Autodesk Inventor part; units mm, degrees
(part 2 of 3)
  spline S217 degree 2 poles (-31.2508, 23.9795) (-31.8051, 23.9795) (-32.4202, 24.6213) (-32.4202, 25.1805) knots 0 0 0 1 2 2 2
  spline S218 degree 2 poles (-32.4202, 25.1805) (-32.4202, 25.7445) (-31.8051, 26.3839) (-31.2508, 26.3839) knots 0 0 0 1 2 2 2
  spline S219 degree 2 poles (-31.2508, 26.3839) (-30.6965, 26.3839) (-30.0839, 25.7421) (-30.0839, 25.1805) knots 0 0 0 1 2 2 2
  spline S220 degree 2 poles (-30.8059, 25.1756) (-30.8059, 25.3774) (-30.8716, 25.6472) (-30.9299, 25.7275) knots 0 0 0 1 2 2 2
  spline S221 degree 2 poles (-30.9299, 25.7275) (-30.9931, 25.8126) (-31.1511, 25.8782) (-31.2508, 25.8782) knots 0 0 0 1 2 2 2
  spline S222 degree 2 poles (-31.2508, 25.8782) (-31.3481, 25.8782) (-31.5012, 25.8199) (-31.5644, 25.7372) knots 0 0 0 1 2 2 2
  spline S223 degree 2 poles (-31.5644, 25.7372) (-31.6252, 25.6594) (-31.6981, 25.3847) (-31.6981, 25.1756) knots 0 0 0 1 2 2 2
  spline S224 degree 2 poles (-31.6981, 25.1756) (-31.6981, 24.969) (-31.6301, 24.7137) (-31.5741, 24.6359) knots 0 0 0 1 2 2 2
  spline S225 degree 2 poles (-31.5741, 24.6359) (-31.5182, 24.5581) (-31.3481, 24.4852) (-31.2459, 24.4852) knots 0 0 0 1 2 2 2
  spline S226 degree 2 poles (-31.2459, 24.4852) (-31.1609, 24.4852) (-30.9858, 24.5581) (-30.9323, 24.631) knots 0 0 0 1 2 2 2
  spline S227 degree 2 poles (-30.9323, 24.631) (-30.8716, 24.7161) (-30.8059, 24.9617) (-30.8059, 25.1756) knots 0 0 0 1 2 2 2
  line L287 (-29.0045, 24.05) -> (-29.7095, 24.05)
  line L288 (-29.7095, 24.05) -> (-29.7095, 27.1837)
  line L289 (-29.7095, 27.1837) -> (-29.0045, 27.1837)
  line L290 (-29.0045, 27.1837) -> (-29.0045, 24.05)
  line L291 (15.1937, 24.05) -> (14.4449, 24.05)
  line L292 (14.4449, 24.05) -> (14.4449, 26.0387)
  line L293 (14.4449, 26.0387) -> (13.9003, 24.755)
  line L294 (13.9003, 24.755) -> (13.3849, 24.755)
  line L295 (13.3849, 24.755) -> (12.8404, 26.0387)
  line L296 (12.8404, 26.0387) -> (12.8404, 24.05)
  line L297 (12.8404, 24.05) -> (12.1305, 24.05)
  line L298 (12.1305, 24.05) -> (12.1305, 27.05)
  line L299 (12.1305, 27.05) -> (12.9984, 27.05)
  line L300 (12.9984, 27.05) -> (13.6645, 25.5694)
  line L301 (13.6645, 25.5694) -> (14.3258, 27.05)
  line L302 (14.3258, 27.05) -> (15.1937, 27.05)
  line L303 (15.1937, 27.05) -> (15.1937, 24.05)
  spline S228 degree 2 poles (17.9457, 25.1805) (17.9457, 24.6213) (17.3355, 23.9795) (16.7788, 23.9795) knots 0 0 0 1 2 2 2
  spline S229 degree 2 poles (16.7788, 23.9795) (16.2245, 23.9795) (15.6094, 24.6213) (15.6094, 25.1805) knots 0 0 0 1 2 2 2
  spline S230 degree 2 poles (15.6094, 25.1805) (15.6094, 25.7445) (16.2245, 26.3839) (16.7788, 26.3839) knots 0 0 0 1 2 2 2
  spline S231 degree 2 poles (16.7788, 26.3839) (17.3331, 26.3839) (17.9457, 25.7421) (17.9457, 25.1805) knots 0 0 0 1 2 2 2
  spline S232 degree 2 poles (17.2237, 25.1756) (17.2237, 25.3774) (17.158, 25.6472) (17.0997, 25.7275) knots 0 0 0 1 2 2 2
  spline S233 degree 2 poles (17.0997, 25.7275) (17.0365, 25.8126) (16.8784, 25.8782) (16.7788, 25.8782) knots 0 0 0 1 2 2 2
  spline S234 degree 2 poles (16.7788, 25.8782) (16.6815, 25.8782) (16.5284, 25.8199) (16.4652, 25.7372) knots 0 0 0 1 2 2 2
  spline S235 degree 2 poles (16.4652, 25.7372) (16.4044, 25.6594) (16.3314, 25.3847) (16.3314, 25.1756) knots 0 0 0 1 2 2 2
  spline S236 degree 2 poles (16.3314, 25.1756) (16.3314, 24.969) (16.3995, 24.7137) (16.4554, 24.6359) knots 0 0 0 1 2 2 2
  spline S237 degree 2 poles (16.4554, 24.6359) (16.5113, 24.5581) (16.6815, 24.4852) (16.7836, 24.4852) knots 0 0 0 1 2 2 2
  spline S238 degree 2 poles (16.7836, 24.4852) (16.8687, 24.4852) (17.0438, 24.5581) (17.0972, 24.631) knots 0 0 0 1 2 2 2
  spline S239 degree 2 poles (17.0972, 24.631) (17.158, 24.7161) (17.2237, 24.9617) (17.2237, 25.1756) knots 0 0 0 1 2 2 2
  spline S240 degree 2 poles (19.1856, 24.0062) (18.7553, 24.0062) (18.3614, 24.3612) (18.3614, 24.7647) knots 0 0 0 1 2 2 2
  line L304 (18.3614, 24.7647) -> (18.3614, 25.8223)
  line L305 (18.3614, 25.8223) -> (18.0916, 25.8223)
  line L306 (18.0916, 25.8223) -> (18.0916, 26.3134)
  line L307 (18.0916, 26.3134) -> (18.3614, 26.3134)
  line L308 (18.3614, 26.3134) -> (18.3614, 26.96)
  line L309 (18.3614, 26.96) -> (19.0665, 26.96)
  line L310 (19.0665, 26.96) -> (19.0665, 26.3134)
  line L311 (19.0665, 26.3134) -> (19.7472, 26.3134)
  line L312 (19.7472, 26.3134) -> (19.7472, 25.8223)
  line L313 (19.7472, 25.8223) -> (19.0665, 25.8223)
  line L314 (19.0665, 25.8223) -> (19.0665, 25.0176)
  spline S241 degree 2 poles (19.0665, 25.0176) (19.0665, 24.8985) (19.0713, 24.721) (19.1005, 24.6505) knots 0 0 0 1 2 2 2
  spline S242 degree 2 poles (19.1005, 24.6505) (19.1297, 24.58) (19.2731, 24.4973) (19.4092, 24.4973) knots 0 0 0 1 2 2 2
  spline S243 degree 2 poles (19.4092, 24.4973) (19.4676, 24.4973) (19.6499, 24.5459) (19.6864, 24.5654) knots 0 0 0 1 2 2 2
  line L315 (19.6864, 24.5654) -> (19.7472, 24.5654)
  line L316 (19.7472, 24.5654) -> (19.7472, 24.0694)
  spline S244 degree 2 poles (19.7472, 24.0694) (19.6329, 24.0403) (19.3752, 24.0062) (19.1856, 24.0062) knots 0 0 0 1 2 2 2
  spline S245 degree 2 poles (22.205, 25.1805) (22.205, 24.6213) (21.5948, 23.9795) (21.0381, 23.9795) knots 0 0 0 1 2 2 2
  spline S246 degree 2 poles (21.0381, 23.9795) (20.4838, 23.9795) (19.8687, 24.6213) (19.8687, 25.1805) knots 0 0 0 1 2 2 2
  spline S247 degree 2 poles (19.8687, 25.1805) (19.8687, 25.7445) (20.4838, 26.3839) (21.0381, 26.3839) knots 0 0 0 1 2 2 2
  spline S248 degree 2 poles (21.0381, 26.3839) (21.5924, 26.3839) (22.205, 25.7421) (22.205, 25.1805) knots 0 0 0 1 2 2 2
  spline S249 degree 2 poles (21.483, 25.1756) (21.483, 25.3774) (21.4173, 25.6472) (21.359, 25.7275) knots 0 0 0 1 2 2 2
  spline S250 degree 2 poles (21.359, 25.7275) (21.2958, 25.8126) (21.1378, 25.8782) (21.0381, 25.8782) knots 0 0 0 1 2 2 2
  spline S251 degree 2 poles (21.0381, 25.8782) (20.9408, 25.8782) (20.7877, 25.8199) (20.7245, 25.7372) knots 0 0 0 1 2 2 2
  spline S252 degree 2 poles (20.7245, 25.7372) (20.6637, 25.6594) (20.5908, 25.3847) (20.5908, 25.1756) knots 0 0 0 1 2 2 2
  spline S253 degree 2 poles (20.5908, 25.1756) (20.5908, 24.969) (20.6588, 24.7137) (20.7147, 24.6359) knots 0 0 0 1 2 2 2
  spline S254 degree 2 poles (20.7147, 24.6359) (20.7707, 24.5581) (20.9408, 24.4852) (21.043, 24.4852) knots 0 0 0 1 2 2 2
  spline S255 degree 2 poles (21.043, 24.4852) (21.128, 24.4852) (21.3031, 24.5581) (21.3566, 24.631) knots 0 0 0 1 2 2 2
  spline S256 degree 2 poles (21.3566, 24.631) (21.4173, 24.7161) (21.483, 24.9617) (21.483, 25.1756) knots 0 0 0 1 2 2 2
  line L317 (24.0989, 25.6448) -> (24.0405, 25.6448)
  spline S257 degree 2 poles (24.0405, 25.6448) (23.9992, 25.6594) (23.846, 25.674) (23.7536, 25.674) knots 0 0 0 1 2 2 2
  spline S258 degree 2 poles (23.7536, 25.674) (23.6442, 25.674) (23.3987, 25.6083) (23.2844, 25.5646) knots 0 0 0 1 2 2 2
  line L318 (23.2844, 25.5646) -> (23.2844, 24.05)
  line L319 (23.2844, 24.05) -> (22.5794, 24.05)
  line L320 (22.5794, 24.05) -> (22.5794, 26.3134)
  line L321 (22.5794, 26.3134) -> (23.2844, 26.3134)
  line L322 (23.2844, 26.3134) -> (23.2844, 25.9876)
  spline S259 degree 2 poles (23.2844, 25.9876) (23.3331, 26.0314) (23.5032, 26.1675) (23.5737, 26.2088) knots 0 0 0 1 2 2 2
  spline S260 degree 2 poles (23.5737, 26.2088) (23.6515, 26.255) (23.8558, 26.3207) (23.9457, 26.3207) knots 0 0 0 1 2 2 2
  spline S261 degree 2 poles (23.9457, 26.3207) (23.9797, 26.3207) (24.0648, 26.3158) (24.0989, 26.3134) knots 0 0 0 1 2 2 2
  line L323 (24.0989, 26.3134) -> (24.0989, 25.6448)
  line L324 (28.1564, 24.05) -> (27.2861, 24.05)
  line L325 (27.2861, 24.05) -> (26.7075, 25.0054)
  line L326 (26.7075, 25.0054) -> (26.1167, 24.05)
  line L327 (26.1167, 24.05) -> (25.2828, 24.05)
  line L328 (25.2828, 24.05) -> (26.2577, 25.5597)
  line L329 (26.2577, 25.5597) -> (25.3217, 27.05)
  line L330 (25.3217, 27.05) -> (26.1921, 27.05)
  line L331 (26.1921, 27.05) -> (26.7342, 26.1432)
  line L332 (26.7342, 26.1432) -> (27.2909, 27.05)
  line L333 (27.2909, 27.05) -> (28.1248, 27.05)
  line L334 (28.1248, 27.05) -> (27.184, 25.5913)
  line L335 (27.184, 25.5913) -> (28.1564, 24.05)
  line L336 (55.2095, 24.05) -> (54.4607, 24.05)
  line L337 (54.4607, 24.05) -> (54.4607, 26.0387)
  line L338 (54.4607, 26.0387) -> (53.9161, 24.755)
  line L339 (53.9161, 24.755) -> (53.4007, 24.755)
  line L340 (53.4007, 24.755) -> (52.8562, 26.0387)
  line L341 (52.8562, 26.0387) -> (52.8562, 24.05)
  line L342 (52.8562, 24.05) -> (52.1463, 24.05)
  line L343 (52.1463, 24.05) -> (52.1463, 27.05)
  line L344 (52.1463, 27.05) -> (53.0142, 27.05)
  line L345 (53.0142, 27.05) -> (53.6803, 25.5694)
  line L346 (53.6803, 25.5694) -> (54.3416, 27.05)
  line L347 (54.3416, 27.05) -> (55.2095, 27.05)
  line L348 (55.2095, 27.05) -> (55.2095, 24.05)
  spline S262 degree 2 poles (57.9615, 25.1805) (57.9615, 24.6213) (57.3513, 23.9795) (56.7946, 23.9795) knots 0 0 0 1 2 2 2
  spline S263 degree 2 poles (56.7946, 23.9795) (56.2403, 23.9795) (55.6252, 24.6213) (55.6252, 25.1805) knots 0 0 0 1 2 2 2
  spline S264 degree 2 poles (55.6252, 25.1805) (55.6252, 25.7445) (56.2403, 26.3839) (56.7946, 26.3839) knots 0 0 0 1 2 2 2
  spline S265 degree 2 poles (56.7946, 26.3839) (57.3489, 26.3839) (57.9615, 25.7421) (57.9615, 25.1805) knots 0 0 0 1 2 2 2
  spline S266 degree 2 poles (57.2395, 25.1756) (57.2395, 25.3774) (57.1738, 25.6472) (57.1155, 25.7275) knots 0 0 0 1 2 2 2
  spline S267 degree 2 poles (57.1155, 25.7275) (57.0523, 25.8126) (56.8942, 25.8782) (56.7946, 25.8782) knots 0 0 0 1 2 2 2
  spline S268 degree 2 poles (56.7946, 25.8782) (56.6973, 25.8782) (56.5442, 25.8199) (56.481, 25.7372) knots 0 0 0 1 2 2 2
  spline S269 degree 2 poles (56.481, 25.7372) (56.4202, 25.6594) (56.3472, 25.3847) (56.3472, 25.1756) knots 0 0 0 1 2 2 2
  spline S270 degree 2 poles (56.3472, 25.1756) (56.3472, 24.969) (56.4153, 24.7137) (56.4712, 24.6359) knots 0 0 0 1 2 2 2
  spline S271 degree 2 poles (56.4712, 24.6359) (56.5271, 24.5581) (56.6973, 24.4852) (56.7994, 24.4852) knots 0 0 0 1 2 2 2
  spline S272 degree 2 poles (56.7994, 24.4852) (56.8845, 24.4852) (57.0596, 24.5581) (57.113, 24.631) knots 0 0 0 1 2 2 2
  spline S273 degree 2 poles (57.113, 24.631) (57.1738, 24.7161) (57.2395, 24.9617) (57.2395, 25.1756) knots 0 0 0 1 2 2 2
  spline S274 degree 2 poles (59.2014, 24.0062) (58.7711, 24.0062) (58.3772, 24.3612) (58.3772, 24.7647) knots 0 0 0 1 2 2 2
  line L349 (58.3772, 24.7647) -> (58.3772, 25.8223)
  line L350 (58.3772, 25.8223) -> (58.1074, 25.8223)
  line L351 (58.1074, 25.8223) -> (58.1074, 26.3134)
  line L352 (58.1074, 26.3134) -> (58.3772, 26.3134)
  line L353 (58.3772, 26.3134) -> (58.3772, 26.96)
  line L354 (58.3772, 26.96) -> (59.0823, 26.96)
  line L355 (59.0823, 26.96) -> (59.0823, 26.3134)
  line L356 (59.0823, 26.3134) -> (59.763, 26.3134)
  line L357 (59.763, 26.3134) -> (59.763, 25.8223)
  line L358 (59.763, 25.8223) -> (59.0823, 25.8223)
  line L359 (59.0823, 25.8223) -> (59.0823, 25.0176)
  spline S275 degree 2 poles (59.0823, 25.0176) (59.0823, 24.8985) (59.0871, 24.721) (59.1163, 24.6505) knots 0 0 0 1 2 2 2
  spline S276 degree 2 poles (59.1163, 24.6505) (59.1455, 24.58) (59.2889, 24.4973) (59.425, 24.4973) knots 0 0 0 1 2 2 2
  spline S277 degree 2 poles (59.425, 24.4973) (59.4834, 24.4973) (59.6657, 24.5459) (59.7022, 24.5654) knots 0 0 0 1 2 2 2
  line L360 (59.7022, 24.5654) -> (59.763, 24.5654)
  line L361 (59.763, 24.5654) -> (59.763, 24.0694)
  spline S278 degree 2 poles (59.763, 24.0694) (59.6487, 24.0403) (59.391, 24.0062) (59.2014, 24.0062) knots 0 0 0 1 2 2 2
  spline S279 degree 2 poles (62.2208, 25.1805) (62.2208, 24.6213) (61.6106, 23.9795) (61.0539, 23.9795) knots 0 0 0 1 2 2 2
  spline S280 degree 2 poles (61.0539, 23.9795) (60.4996, 23.9795) (59.8845, 24.6213) (59.8845, 25.1805) knots 0 0 0 1 2 2 2
  spline S281 degree 2 poles (59.8845, 25.1805) (59.8845, 25.7445) (60.4996, 26.3839) (61.0539, 26.3839) knots 0 0 0 1 2 2 2
  spline S282 degree 2 poles (61.0539, 26.3839) (61.6082, 26.3839) (62.2208, 25.7421) (62.2208, 25.1805) knots 0 0 0 1 2 2 2
  spline S283 degree 2 poles (61.4988, 25.1756) (61.4988, 25.3774) (61.4331, 25.6472) (61.3748, 25.7275) knots 0 0 0 1 2 2 2
  spline S284 degree 2 poles (61.3748, 25.7275) (61.3116, 25.8126) (61.1536, 25.8782) (61.0539, 25.8782) knots 0 0 0 1 2 2 2
  spline S285 degree 2 poles (61.0539, 25.8782) (60.9566, 25.8782) (60.8035, 25.8199) (60.7403, 25.7372) knots 0 0 0 1 2 2 2
  spline S286 degree 2 poles (60.7403, 25.7372) (60.6795, 25.6594) (60.6066, 25.3847) (60.6066, 25.1756) knots 0 0 0 1 2 2 2
  spline S287 degree 2 poles (60.6066, 25.1756) (60.6066, 24.969) (60.6746, 24.7137) (60.7306, 24.6359) knots 0 0 0 1 2 2 2
  spline S288 degree 2 poles (60.7306, 24.6359) (60.7865, 24.5581) (60.9566, 24.4852) (61.0588, 24.4852) knots 0 0 0 1 2 2 2
  spline S289 degree 2 poles (61.0588, 24.4852) (61.1438, 24.4852) (61.3189, 24.5581) (61.3724, 24.631) knots 0 0 0 1 2 2 2
  spline S290 degree 2 poles (61.3724, 24.631) (61.4331, 24.7161) (61.4988, 24.9617) (61.4988, 25.1756) knots 0 0 0 1 2 2 2
  line L362 (64.1147, 25.6448) -> (64.0563, 25.6448)
  spline S291 degree 2 poles (64.0563, 25.6448) (64.015, 25.6594) (63.8618, 25.674) (63.7694, 25.674) knots 0 0 0 1 2 2 2
  spline S292 degree 2 poles (63.7694, 25.674) (63.66, 25.674) (63.4145, 25.6083) (63.3002, 25.5646) knots 0 0 0 1 2 2 2
  line L363 (63.3002, 25.5646) -> (63.3002, 24.05)
  line L364 (63.3002, 24.05) -> (62.5952, 24.05)
  line L365 (62.5952, 24.05) -> (62.5952, 26.3134)
  line L366 (62.5952, 26.3134) -> (63.3002, 26.3134)
  line L367 (63.3002, 26.3134) -> (63.3002, 25.9876)
  spline S293 degree 2 poles (63.3002, 25.9876) (63.3489, 26.0314) (63.519, 26.1675) (63.5895, 26.2088) knots 0 0 0 1 2 2 2
  spline S294 degree 2 poles (63.5895, 26.2088) (63.6673, 26.255) (63.8716, 26.3207) (63.9615, 26.3207) knots 0 0 0 1 2 2 2
  spline S295 degree 2 poles (63.9615, 26.3207) (63.9955, 26.3207) (64.0806, 26.3158) (64.1147, 26.3134) knots 0 0 0 1 2 2 2
  line L368 (64.1147, 26.3134) -> (64.1147, 25.6448)
  line L369 (68.1284, 27.05) -> (67.0928, 25.302)
  line L370 (67.0928, 25.302) -> (67.0928, 24.05)
  line L371 (67.0928, 24.05) -> (66.3391, 24.05)
  line L372 (66.3391, 24.05) -> (66.3391, 25.2656)
  line L373 (66.3391, 25.2656) -> (65.2865, 27.05)
  line L374 (65.2865, 27.05) -> (66.1447, 27.05)
  line L375 (66.1447, 27.05) -> (66.7306, 25.9803)
  line L376 (66.7306, 25.9803) -> (67.297, 27.05)
  line L377 (67.297, 27.05) -> (68.1284, 27.05)
  line L378 (95.3468, 24.05) -> (94.5981, 24.05)
  line L379 (94.5981, 24.05) -> (94.5981, 26.0387)
  line L380 (94.5981, 26.0387) -> (94.0535, 24.755)
  line L381 (94.0535, 24.755) -> (93.5381, 24.755)
  line L382 (93.5381, 24.755) -> (92.9935, 26.0387)
  line L383 (92.9935, 26.0387) -> (92.9935, 24.05)
  line L384 (92.9935, 24.05) -> (92.2836, 24.05)
  line L385 (92.2836, 24.05) -> (92.2836, 27.05)
  line L386 (92.2836, 27.05) -> (93.1515, 27.05)
  line L387 (93.1515, 27.05) -> (93.8177, 25.5694)
  line L388 (93.8177, 25.5694) -> (94.4789, 27.05)
  line L389 (94.4789, 27.05) -> (95.3468, 27.05)
  line L390 (95.3468, 27.05) -> (95.3468, 24.05)
  spline S296 degree 2 poles (98.0989, 25.1805) (98.0989, 24.6213) (97.4887, 23.9795) (96.9319, 23.9795) knots 0 0 0 1 2 2 2
  spline S297 degree 2 poles (96.9319, 23.9795) (96.3776, 23.9795) (95.7626, 24.6213) (95.7626, 25.1805) knots 0 0 0 1 2 2 2
  spline S298 degree 2 poles (95.7626, 25.1805) (95.7626, 25.7445) (96.3776, 26.3839) (96.9319, 26.3839) knots 0 0 0 1 2 2 2
  spline S299 degree 2 poles (96.9319, 26.3839) (97.4862, 26.3839) (98.0989, 25.7421) (98.0989, 25.1805) knots 0 0 0 1 2 2 2
  spline S300 degree 2 poles (97.3768, 25.1756) (97.3768, 25.3774) (97.3112, 25.6472) (97.2528, 25.7275) knots 0 0 0 1 2 2 2
  spline S301 degree 2 poles (97.2528, 25.7275) (97.1896, 25.8126) (97.0316, 25.8782) (96.9319, 25.8782) knots 0 0 0 1 2 2 2
  spline S302 degree 2 poles (96.9319, 25.8782) (96.8347, 25.8782) (96.6815, 25.8199) (96.6183, 25.7372) knots 0 0 0 1 2 2 2
  spline S303 degree 2 poles (96.6183, 25.7372) (96.5575, 25.6594) (96.4846, 25.3847) (96.4846, 25.1756) knots 0 0 0 1 2 2 2
  spline S304 degree 2 poles (96.4846, 25.1756) (96.4846, 24.969) (96.5527, 24.7137) (96.6086, 24.6359) knots 0 0 0 1 2 2 2
  spline S305 degree 2 poles (96.6086, 24.6359) (96.6645, 24.5581) (96.8347, 24.4852) (96.9368, 24.4852) knots 0 0 0 1 2 2 2
  spline S306 degree 2 poles (96.9368, 24.4852) (97.0219, 24.4852) (97.1969, 24.5581) (97.2504, 24.631) knots 0 0 0 1 2 2 2
  spline S307 degree 2 poles (97.2504, 24.631) (97.3112, 24.7161) (97.3768, 24.9617) (97.3768, 25.1756) knots 0 0 0 1 2 2 2
  spline S308 degree 2 poles (99.3387, 24.0062) (98.9084, 24.0062) (98.5146, 24.3612) (98.5146, 24.7647) knots 0 0 0 1 2 2 2
  line L391 (98.5146, 24.7647) -> (98.5146, 25.8223)
  line L392 (98.5146, 25.8223) -> (98.2447, 25.8223)
  line L393 (98.2447, 25.8223) -> (98.2447, 26.3134)
  line L394 (98.2447, 26.3134) -> (98.5146, 26.3134)
  line L395 (98.5146, 26.3134) -> (98.5146, 26.96)
  line L396 (98.5146, 26.96) -> (99.2196, 26.96)
  line L397 (99.2196, 26.96) -> (99.2196, 26.3134)
  line L398 (99.2196, 26.3134) -> (99.9003, 26.3134)
  line L399 (99.9003, 26.3134) -> (99.9003, 25.8223)
  line L400 (99.9003, 25.8223) -> (99.2196, 25.8223)
  line L401 (99.2196, 25.8223) -> (99.2196, 25.0176)
  spline S309 degree 2 poles (99.2196, 25.0176) (99.2196, 24.8985) (99.2245, 24.721) (99.2536, 24.6505) knots 0 0 0 1 2 2 2
  spline S310 degree 2 poles (99.2536, 24.6505) (99.2828, 24.58) (99.4263, 24.4973) (99.5624, 24.4973) knots 0 0 0 1 2 2 2
  spline S311 degree 2 poles (99.5624, 24.4973) (99.6207, 24.4973) (99.8031, 24.5459) (99.8395, 24.5654) knots 0 0 0 1 2 2 2
  line L402 (99.8395, 24.5654) -> (99.9003, 24.5654)
  line L403 (99.9003, 24.5654) -> (99.9003, 24.0694)
  spline S312 degree 2 poles (99.9003, 24.0694) (99.7861, 24.0403) (99.5284, 24.0062) (99.3387, 24.0062) knots 0 0 0 1 2 2 2
  spline S313 degree 2 poles (102.3582, 25.1805) (102.3582, 24.6213) (101.748, 23.9795) (101.1912, 23.9795) knots 0 0 0 1 2 2 2
  spline S314 degree 2 poles (101.1912, 23.9795) (100.637, 23.9795) (100.0219, 24.6213) (100.0219, 25.1805) knots 0 0 0 1 2 2 2
  spline S315 degree 2 poles (100.0219, 25.1805) (100.0219, 25.7445) (100.637, 26.3839) (101.1912, 26.3839) knots 0 0 0 1 2 2 2
  spline S316 degree 2 poles (101.1912, 26.3839) (101.7455, 26.3839) (102.3582, 25.7421) (102.3582, 25.1805) knots 0 0 0 1 2 2 2
  spline S317 degree 2 poles (101.6361, 25.1756) (101.6361, 25.3774) (101.5705, 25.6472) (101.5122, 25.7275) knots 0 0 0 1 2 2 2
  spline S318 degree 2 poles (101.5122, 25.7275) (101.4489, 25.8126) (101.2909, 25.8782) (101.1912, 25.8782) knots 0 0 0 1 2 2 2
  spline S319 degree 2 poles (101.1912, 25.8782) (101.094, 25.8782) (100.9408, 25.8199) (100.8776, 25.7372) knots 0 0 0 1 2 2 2
  spline S320 degree 2 poles (100.8776, 25.7372) (100.8169, 25.6594) (100.7439, 25.3847) (100.7439, 25.1756) knots 0 0 0 1 2 2 2
  spline S321 degree 2 poles (100.7439, 25.1756) (100.7439, 24.969) (100.812, 24.7137) (100.8679, 24.6359) knots 0 0 0 1 2 2 2
  spline S322 degree 2 poles (100.8679, 24.6359) (100.9238, 24.5581) (101.094, 24.4852) (101.1961, 24.4852) knots 0 0 0 1 2 2 2
  spline S323 degree 2 poles (101.1961, 24.4852) (101.2812, 24.4852) (101.4562, 24.5581) (101.5097, 24.631) knots 0 0 0 1 2 2 2
  spline S324 degree 2 poles (101.5097, 24.631) (101.5705, 24.7161) (101.6361, 24.9617) (101.6361, 25.1756) knots 0 0 0 1 2 2 2
  line L404 (104.252, 25.6448) -> (104.1937, 25.6448)
  spline S325 degree 2 poles (104.1937, 25.6448) (104.1524, 25.6594) (103.9992, 25.674) (103.9068, 25.674) knots 0 0 0 1 2 2 2
  spline S326 degree 2 poles (103.9068, 25.674) (103.7974, 25.674) (103.5519, 25.6083) (103.4376, 25.5646) knots 0 0 0 1 2 2 2
  line L405 (103.4376, 25.5646) -> (103.4376, 24.05)
  line L406 (103.4376, 24.05) -> (102.7326, 24.05)
  line L407 (102.7326, 24.05) -> (102.7326, 26.3134)
  line L408 (102.7326, 26.3134) -> (103.4376, 26.3134)
  line L409 (103.4376, 26.3134) -> (103.4376, 25.9876)
  spline S327 degree 2 poles (103.4376, 25.9876) (103.4862, 26.0314) (103.6564, 26.1675) (103.7269, 26.2088) knots 0 0 0 1 2 2 2
  spline S328 degree 2 poles (103.7269, 26.2088) (103.8047, 26.255) (104.0089, 26.3207) (104.0989, 26.3207) knots 0 0 0 1 2 2 2
  spline S329 degree 2 poles (104.0989, 26.3207) (104.1329, 26.3207) (104.218, 26.3158) (104.252, 26.3134) knots 0 0 0 1 2 2 2
  line L410 (104.252, 26.3134) -> (104.252, 25.6448)
  line L411 (107.9473, 24.05) -> (105.5697, 24.05)
  line L412 (105.5697, 24.05) -> (105.5697, 24.6116)
  line L413 (105.5697, 24.6116) -> (106.953, 26.4787)
  line L414 (106.953, 26.4787) -> (105.6426, 26.4787)
  line L415 (105.6426, 26.4787) -> (105.6426, 27.05)
  line L416 (105.6426, 27.05) -> (107.8671, 27.05)
  line L417 (107.8671, 27.05) -> (107.8671, 26.4787)
  line L418 (107.8671, 26.4787) -> (106.4887, 24.6213)
  line L419 (106.4887, 24.6213) -> (107.9473, 24.6213)
  line L420 (107.9473, 24.6213) -> (107.9473, 24.05)
  spline S330 degree 2 poles (121.0348, 26.1043) (121.0348, 25.8952) (120.9011, 25.516) (120.7771, 25.3895) knots 0 0 0 1 2 2 2
  spline S331 degree 2 poles (120.7771, 25.3895) (120.7018, 25.3093) (120.517, 25.178) (120.4076, 25.1318) knots 0 0 0 1 2 2 2
  spline S332 degree 2 poles (120.4076, 25.1318) (120.2958, 25.0857) (120.0357, 25.0322) (119.8752, 25.0322) knots 0 0 0 1 2 2 2
  line L421 (119.8752, 25.0322) -> (119.4814, 25.0322)
  line L422 (119.4814, 25.0322) -> (119.4814, 24.05)
  line L423 (119.4814, 24.05) -> (118.7277, 24.05)
  line L424 (118.7277, 24.05) -> (118.7277, 27.05)
  line L425 (118.7277, 27.05) -> (119.8922, 27.05)
  spline S333 degree 2 poles (119.8922, 27.05) (120.1499, 27.05) (120.5267, 26.9552) (120.6799, 26.8531) knots 0 0 0 1 2 2 2
  spline S334 degree 2 poles (120.6799, 26.8531) (120.8501, 26.7388) (121.0348, 26.3644) (121.0348, 26.1043) knots 0 0 0 1 2 2 2
  spline S335 degree 2 poles (120.2617, 26.0848) (120.2617, 26.2137) (120.1402, 26.396) (120.0575, 26.4301) knots 0 0 0 1 2 2 2
  spline S336 degree 2 poles (120.0575, 26.4301) (119.9506, 26.4763) (119.7561, 26.4908) (119.5883, 26.4908) knots 0 0 0 1 2 2 2
  line L426 (119.5883, 26.4908) -> (119.4814, 26.4908)
  line L427 (119.4814, 26.4908) -> (119.4814, 25.5913)
  line L428 (119.4814, 25.5913) -> (119.5348, 25.5913)
  spline S337 degree 2 poles (119.5348, 25.5913) (119.6394, 25.5913) (119.829, 25.5962) (119.8995, 25.6083) knots 0 0 0 1 2 2 2
  spline S338 degree 2 poles (119.8995, 25.6083) (119.9603, 25.6181) (120.094, 25.6764) (120.1305, 25.7129) knots 0 0 0 1 2 2 2
  spline S339 degree 2 poles (120.1305, 25.7129) (120.2083, 25.7858) (120.2617, 25.9487) (120.2617, 26.0848) knots 0 0 0 1 2 2 2
  spline S340 degree 2 poles (123.5681, 25.1805) (123.5681, 24.6213) (122.9579, 23.9795) (122.4011, 23.9795) knots 0 0 0 1 2 2 2
  spline S341 degree 2 poles (122.4011, 23.9795) (121.8468, 23.9795) (121.2318, 24.6213) (121.2318, 25.1805) knots 0 0 0 1 2 2 2
  spline S342 degree 2 poles (121.2318, 25.1805) (121.2318, 25.7445) (121.8468, 26.3839) (122.4011, 26.3839) knots 0 0 0 1 2 2 2
  spline S343 degree 2 poles (122.4011, 26.3839) (122.9554, 26.3839) (123.5681, 25.7421) (123.5681, 25.1805) knots 0 0 0 1 2 2 2
  spline S344 degree 2 poles (122.846, 25.1756) (122.846, 25.3774) (122.7804, 25.6472) (122.722, 25.7275) knots 0 0 0 1 2 2 2
  spline S345 degree 2 poles (122.722, 25.7275) (122.6588, 25.8126) (122.5008, 25.8782) (122.4011, 25.8782) knots 0 0 0 1 2 2 2
  spline S346 degree 2 poles (122.4011, 25.8782) (122.3039, 25.8782) (122.1507, 25.8199) (122.0875, 25.7372) knots 0 0 0 1 2 2 2
  spline S347 degree 2 poles (122.0875, 25.7372) (122.0267, 25.6594) (121.9538, 25.3847) (121.9538, 25.1756) knots 0 0 0 1 2 2 2
  spline S348 degree 2 poles (121.9538, 25.1756) (121.9538, 24.969) (122.0219, 24.7137) (122.0778, 24.6359) knots 0 0 0 1 2 2 2
  spline S349 degree 2 poles (122.0778, 24.6359) (122.1337, 24.5581) (122.3039, 24.4852) (122.406, 24.4852) knots 0 0 0 1 2 2 2
  spline S350 degree 2 poles (122.406, 24.4852) (122.4911, 24.4852) (122.6661, 24.5581) (122.7196, 24.631) knots 0 0 0 1 2 2 2
  spline S351 degree 2 poles (122.7196, 24.631) (122.7804, 24.7161) (122.846, 24.9617) (122.846, 25.1756) knots 0 0 0 1 2 2 2
  line L429 (127.3144, 26.3134) -> (126.6532, 24.05)
  line L430 (126.6532, 24.05) -> (125.9044, 24.05)
  line L431 (125.9044, 24.05) -> (125.5057, 25.5135)
  line L432 (125.5057, 25.5135) -> (125.107, 24.05)
  line L433 (125.107, 24.05) -> (124.3582, 24.05)
  line L434 (124.3582, 24.05) -> (123.7018, 26.3134)
  line L435 (123.7018, 26.3134) -> (124.4433, 26.3134)
  line L436 (124.4433, 26.3134) -> (124.7909, 24.8158)
  line L437 (124.7909, 24.8158) -> (125.2188, 26.3134)
  line L438 (125.2188, 26.3134) -> (125.8436, 26.3134)
  line L439 (125.8436, 26.3134) -> (126.2472, 24.8158)
  line L440 (126.2472, 24.8158) -> (126.59, 26.3134)
  line L441 (126.59, 26.3134) -> (127.3144, 26.3134)
  spline S352 degree 2 poles (128.7731, 23.9892) (128.1313, 23.9892) (127.4481, 24.6019) (127.4481, 25.1683) knots 0 0 0 1 2 2 2
  spline S353 degree 2 poles (127.4481, 25.1683) (127.4481, 25.7226) (128.0851, 26.3839) (128.6588, 26.3839) knots 0 0 0 1 2 2 2
  spline S354 degree 2 poles (128.6588, 26.3839) (129.1767, 26.3839) (129.7018, 25.8223) (129.7018, 25.302) knots 0 0 0 1 2 2 2
  line L442 (129.7018, 25.302) -> (129.7018, 25.0468)
  line L443 (129.7018, 25.0468) -> (128.1532, 25.0468)
  spline S355 degree 2 poles (128.1532, 25.0468) (128.1629, 24.8887) (128.2771, 24.6797) (128.3695, 24.6165) knots 0 0 0 1 2 2 2
  spline S356 degree 2 poles (128.3695, 24.6165) (128.4595, 24.5532) (128.7026, 24.4998) (128.846, 24.4998) knots 0 0 0 1 2 2 2
  spline S357 degree 2 poles (128.846, 24.4998) (128.9676, 24.4998) (129.2058, 24.5532) (129.3055, 24.5994) knots 0 0 0 1 2 2 2
  spline S358 degree 2 poles (129.3055, 24.5994) (129.393, 24.6359) (129.5389, 24.7259) (129.5851, 24.7599) knots 0 0 0 1 2 2 2
  line L444 (129.5851, 24.7599) -> (129.6605, 24.7599)
  line L445 (129.6605, 24.7599) -> (129.6605, 24.1764)
  spline S359 degree 2 poles (129.6605, 24.1764) (129.5729, 24.1424) (129.4319, 24.084) (129.3055, 24.0549) knots 0 0 0 1 2 2 2
  spline S360 degree 2 poles (129.3055, 24.0549) (129.1912, 24.0233) (128.9481, 23.9892) (128.7731, 23.9892) knots 0 0 0 1 2 2 2
  spline S361 degree 2 poles (129.0065, 25.4722) (129.0016, 25.6959) (128.8047, 25.9317) (128.6029, 25.9317) knots 0 0 0 1 2 2 2
  spline S362 degree 2 poles (128.6029, 25.9317) (128.3963, 25.9317) (128.1629, 25.6837) (128.1507, 25.4722) knots 0 0 0 1 2 2 2
  line L446 (128.1507, 25.4722) -> (129.0065, 25.4722)
  line L447 (131.5835, 25.6448) -> (131.5251, 25.6448)
  spline S363 degree 2 poles (131.5251, 25.6448) (131.4838, 25.6594) (131.3306, 25.674) (131.2383, 25.674) knots 0 0 0 1 2 2 2
  spline S364 degree 2 poles (131.2383, 25.674) (131.1288, 25.674) (130.8833, 25.6083) (130.769, 25.5646) knots 0 0 0 1 2 2 2
  line L448 (130.769, 25.5646) -> (130.769, 24.05)
  line L449 (130.769, 24.05) -> (130.064, 24.05)
  line L450 (130.064, 24.05) -> (130.064, 26.3134)
  line L451 (130.064, 26.3134) -> (130.769, 26.3134)
  line L452 (130.769, 26.3134) -> (130.769, 25.9876)
  spline S365 degree 2 poles (130.769, 25.9876) (130.8177, 26.0314) (130.9878, 26.1675) (131.0583, 26.2088) knots 0 0 0 1 2 2 2
  spline S366 degree 2 poles (131.0583, 26.2088) (131.1361, 26.255) (131.3404, 26.3207) (131.4303, 26.3207) knots 0 0 0 1 2 2 2
  spline S367 degree 2 poles (131.4303, 26.3207) (131.4643, 26.3207) (131.5494, 26.3158) (131.5835, 26.3134) knots 0 0 0 1 2 2 2
  line L453 (131.5835, 26.3134) -> (131.5835, 25.6448)
  line L454 (140.7472, 24.05) -> (140.7472, 27.55)
  line L455 (140.7472, 27.55) -> (143.1126, 27.55)
  line L456 (143.1126, 27.55) -> (143.1126, 26.8835)
  line L457 (143.1126, 26.8835) -> (141.6207, 26.8835)
  line L458 (141.6207, 26.8835) -> (141.6207, 26.268)
  line L459 (141.6207, 26.268) -> (142.9964, 26.268)
  line L460 (142.9964, 26.268) -> (142.9964, 25.6015)
  line L461 (142.9964, 25.6015) -> (141.6207, 25.6015)
  line L462 (141.6207, 25.6015) -> (141.6207, 24.7165)
  line L463 (141.6207, 24.7165) -> (143.1126, 24.7165)
  line L464 (143.1126, 24.7165) -> (143.1126, 24.05)
  line L465 (143.1126, 24.05) -> (140.7472, 24.05)
  line L466 (146.8112, 24.05) -> (146.8112, 25.3689)
  spline S368 degree 2 poles (146.8112, 25.3689) (146.8112, 25.5646) (146.797, 25.8312) (146.763, 25.9163) knots 0 0 0 1 2 2 2
  spline S369 degree 2 poles (146.763, 25.9163) (146.7261, 26.0014) (146.5786, 26.078) (146.4453, 26.078) knots 0 0 0 1 2 2 2
  spline S370 degree 2 poles (146.4453, 26.078) (146.3517, 26.078) (146.1702, 25.9957) (146.0624, 25.9191) knots 0 0 0 1 2 2 2
  line L467 (146.0624, 25.9191) -> (146.0624, 24.05)
  line L468 (146.0624, 24.05) -> (145.2342, 24.05)
  line L469 (145.2342, 24.05) -> (145.2342, 25.3689)
  spline S371 degree 2 poles (145.2342, 25.3689) (145.2342, 25.5618) (145.2172, 25.8312) (145.1831, 25.9163) knots 0 0 0 1 2 2 2
  spline S372 degree 2 poles (145.1831, 25.9163) (145.1463, 26.0014) (144.9988, 26.078) (144.8655, 26.078) knots 0 0 0 1 2 2 2
  spline S373 degree 2 poles (144.8655, 26.078) (144.7662, 26.078) (144.5705, 25.9844) (144.4797, 25.9191) knots 0 0 0 1 2 2 2
  line L470 (144.4797, 25.9191) -> (144.4797, 24.05)
  line L471 (144.4797, 24.05) -> (143.6572, 24.05)
  line L472 (143.6572, 24.05) -> (143.6572, 26.6906)
  line L473 (143.6572, 26.6906) -> (144.4797, 26.6906)
  line L474 (144.4797, 26.6906) -> (144.4797, 26.3985)
  spline S374 degree 2 poles (144.4797, 26.3985) (144.6811, 26.5686) (145.0413, 26.7615) (145.2654, 26.7615) knots 0 0 0 1 2 2 2
  spline S375 degree 2 poles (145.2654, 26.7615) (145.5065, 26.7615) (145.8752, 26.5318) (145.9716, 26.302) knots 0 0 0 1 2 2 2
  spline S376 degree 2 poles (145.9716, 26.302) (146.207, 26.5233) (146.6268, 26.7615) (146.8424, 26.7615) knots 0 0 0 1 2 2 2
  spline S377 degree 2 poles (146.8424, 26.7615) (147.0267, 26.7615) (147.3189, 26.6452) (147.4182, 26.5261) knots 0 0 0 1 2 2 2
  spline S378 degree 2 poles (147.4182, 26.5261) (147.5288, 26.3985) (147.6394, 26.0496) (147.6394, 25.7688) knots 0 0 0 1 2 2 2
  line L475 (147.6394, 25.7688) -> (147.6394, 24.05)
  line L476 (147.6394, 24.05) -> (146.8112, 24.05)
  spline S379 degree 2 poles (149.6021, 23.9791) (148.8533, 23.9791) (148.0563, 24.6938) (148.0563, 25.3547) knots 0 0 0 1 2 2 2
  spline S380 degree 2 poles (148.0563, 25.3547) (148.0563, 26.0014) (148.7994, 26.7729) (149.4688, 26.7729) knots 0 0 0 1 2 2 2
  spline S381 degree 2 poles (149.4688, 26.7729) (150.0729, 26.7729) (150.6856, 26.1177) (150.6856, 25.5107) knots 0 0 0 1 2 2 2
  line L477 (150.6856, 25.5107) -> (150.6856, 25.2129)
  line L478 (150.6856, 25.2129) -> (148.8788, 25.2129)
  spline S382 degree 2 poles (148.8788, 25.2129) (148.8902, 25.0285) (149.0235, 24.7846) (149.1313, 24.7109) knots 0 0 0 1 2 2 2
  spline S383 degree 2 poles (149.1313, 24.7109) (149.2362, 24.6371) (149.5199, 24.5747) (149.6872, 24.5747) knots 0 0 0 1 2 2 2
  spline S384 degree 2 poles (149.6872, 24.5747) (149.829, 24.5747) (150.107, 24.6371) (150.2233, 24.691) knots 0 0 0 1 2 2 2
  spline S385 degree 2 poles (150.2233, 24.691) (150.3254, 24.7335) (150.4955, 24.8385) (150.5494, 24.8782) knots 0 0 0 1 2 2 2
  line L479 (150.5494, 24.8782) -> (150.6374, 24.8782)
  line L480 (150.6374, 24.8782) -> (150.6374, 24.1975)
  spline S386 degree 2 poles (150.6374, 24.1975) (150.5353, 24.1578) (150.3707, 24.0897) (150.2233, 24.0557) knots 0 0 0 1 2 2 2
  spline S387 degree 2 poles (150.2233, 24.0557) (150.09, 24.0188) (149.8063, 23.9791) (149.6021, 23.9791) knots 0 0 0 1 2 2 2
  spline S388 degree 2 poles (149.8744, 25.7092) (149.8687, 25.9702) (149.639, 26.2453) (149.4036, 26.2453) knots 0 0 0 1 2 2 2
  spline S389 degree 2 poles (149.4036, 26.2453) (149.1625, 26.2453) (148.8902, 25.956) (148.876, 25.7092) knots 0 0 0 1 2 2 2
  line L481 (148.876, 25.7092) -> (149.8744, 25.7092)
  line L482 (152.8809, 25.9106) -> (152.8128, 25.9106)
  spline S390 degree 2 poles (152.8128, 25.9106) (152.7646, 25.9276) (152.5859, 25.9447) (152.4781, 25.9447) knots 0 0 0 1 2 2 2
  spline S391 degree 2 poles (152.4781, 25.9447) (152.3505, 25.9447) (152.064, 25.8681) (151.9307, 25.817) knots 0 0 0 1 2 2 2
  line L483 (151.9307, 25.817) -> (151.9307, 24.05)
  line L484 (151.9307, 24.05) -> (151.1082, 24.05)
  line L485 (151.1082, 24.05) -> (151.1082, 26.6906)
  line L486 (151.1082, 26.6906) -> (151.9307, 26.6906)
  line L487 (151.9307, 26.6906) -> (151.9307, 26.3105)
  spline S392 degree 2 poles (151.9307, 26.3105) (151.9874, 26.3616) (152.186, 26.5204) (152.2682, 26.5686) knots 0 0 0 1 2 2 2
  spline S393 degree 2 poles (152.2682, 26.5686) (152.359, 26.6225) (152.5972, 26.6991) (152.7022, 26.6991) knots 0 0 0 1 2 2 2
  spline S394 degree 2 poles (152.7022, 26.6991) (152.7419, 26.6991) (152.8412, 26.6934) (152.8809, 26.6906) knots 0 0 0 1 2 2 2
  line L488 (152.8809, 26.6906) -> (152.8809, 25.9106)
  spline S395 degree 2 poles (155.5952, 24.3535) (155.5952, 23.9876) (155.3825, 23.4742) (155.201, 23.3324) knots 0 0 0 1 2 2 2
  spline S396 degree 2 poles (155.201, 23.3324) (155.0166, 23.1878) (154.5061, 23.0573) (154.1941, 23.0573) knots 0 0 0 1 2 2 2
  spline S397 degree 2 poles (154.1941, 23.0573) (153.9303, 23.0573) (153.4566, 23.1254) (153.2836, 23.1707) knots 0 0 0 1 2 2 2
  line L489 (153.2836, 23.1707) -> (153.2836, 23.8316)
  line L490 (153.2836, 23.8316) -> (153.3801, 23.8316)
  spline S398 degree 2 poles (153.3801, 23.8316) (153.4396, 23.8089) (153.607, 23.7522) (153.6921, 23.7295) knots 0 0 0 1 2 2 2
  spline S399 degree 2 poles (153.6921, 23.7295) (153.7942, 23.704) (153.987, 23.6699) (154.0863, 23.6699) knots 0 0 0 1 2 2 2
  spline S400 degree 2 poles (154.0863, 23.6699) (154.2962, 23.6699) (154.5741, 23.755) (154.6451, 23.8344) knots 0 0 0 1 2 2 2
  spline S401 degree 2 poles (154.6451, 23.8344) (154.716, 23.9167) (154.7727, 24.1379) (154.7727, 24.3081) knots 0 0 0 1 2 2 2
  line L491 (154.7727, 24.3081) -> (154.7727, 24.3563)
  spline S402 degree 2 poles (154.7727, 24.3563) (154.6337, 24.2344) (154.2707, 24.0869) (154.0778, 24.0869) knots 0 0 0 1 2 2 2
  spline S403 degree 2 poles (154.0778, 24.0869) (153.5644, 24.0869) (153.0085, 24.7534) (153.0085, 25.437) knots 0 0 0 1 2 2 2
  spline S404 degree 2 poles (153.0085, 25.437) (153.0085, 25.7461) (153.1787, 26.2396) (153.3318, 26.4126) knots 0 0 0 1 2 2 2
  spline S405 degree 2 poles (153.3318, 26.4126) (153.4793, 26.58) (153.8906, 26.7615) (154.1147, 26.7615) knots 0 0 0 1 2 2 2
  spline S406 degree 2 poles (154.1147, 26.7615) (154.316, 26.7615) (154.6365, 26.6594) (154.767, 26.5743) knots 0 0 0 1 2 2 2
  line L492 (154.767, 26.5743) -> (154.7982, 26.6906)
  line L493 (154.7982, 26.6906) -> (155.5952, 26.6906)
  line L494 (155.5952, 26.6906) -> (155.5952, 24.3535)
  line L495 (154.7727, 24.881) -> (154.7727, 26.078)
  spline S407 degree 2 poles (154.7727, 26.078) (154.7131, 26.1063) (154.5344, 26.1432) (154.4437, 26.1432) knots 0 0 0 1 2 2 2
  spline S408 degree 2 poles (154.4437, 26.1432) (154.1487, 26.1432) (153.8509, 25.7603) (153.8509, 25.4171) knots 0 0 0 1 2 2 2
  spline S409 degree 2 poles (153.8509, 25.4171) (153.8509, 25.2469) (153.8963, 25.0087) (153.9558, 24.9179) knots 0 0 0 1 2 2 2
  spline S410 degree 2 poles (153.9558, 24.9179) (154.0154, 24.8271) (154.2054, 24.7364) (154.3529, 24.7364) knots 0 0 0 1 2 2 2
  spline S411 degree 2 poles (154.3529, 24.7364) (154.4635, 24.7364) (154.6763, 24.813) (154.7727, 24.881) knots 0 0 0 1 2 2 2
  spline S412 degree 2 poles (157.5778, 23.9791) (156.829, 23.9791) (156.032, 24.6938) (156.032, 25.3547) knots 0 0 0 1 2 2 2
  spline S413 degree 2 poles (156.032, 25.3547) (156.032, 26.0014) (156.7751, 26.7729) (157.4445, 26.7729) knots 0 0 0 1 2 2 2
  spline S414 degree 2 poles (157.4445, 26.7729) (158.0486, 26.7729) (158.6613, 26.1177) (158.6613, 25.5107) knots 0 0 0 1 2 2 2
  line L496 (158.6613, 25.5107) -> (158.6613, 25.2129)
  line L497 (158.6613, 25.2129) -> (156.8545, 25.2129)
  spline S415 degree 2 poles (156.8545, 25.2129) (156.8659, 25.0285) (156.9992, 24.7846) (157.107, 24.7109) knots 0 0 0 1 2 2 2
  spline S416 degree 2 poles (157.107, 24.7109) (157.2119, 24.6371) (157.4955, 24.5747) (157.6629, 24.5747) knots 0 0 0 1 2 2 2
  spline S417 degree 2 poles (157.6629, 24.5747) (157.8047, 24.5747) (158.0827, 24.6371) (158.1989, 24.691) knots 0 0 0 1 2 2 2
  spline S418 degree 2 poles (158.1989, 24.691) (158.3011, 24.7335) (158.4712, 24.8385) (158.5251, 24.8782) knots 0 0 0 1 2 2 2
  line L498 (158.5251, 24.8782) -> (158.613, 24.8782)
  line L499 (158.613, 24.8782) -> (158.613, 24.1975)
  spline S419 degree 2 poles (158.613, 24.1975) (158.5109, 24.1578) (158.3464, 24.0897) (158.1989, 24.0557) knots 0 0 0 1 2 2 2
  spline S420 degree 2 poles (158.1989, 24.0557) (158.0656, 24.0188) (157.782, 23.9791) (157.5778, 23.9791) knots 0 0 0 1 2 2 2
  spline S421 degree 2 poles (157.8501, 25.7092) (157.8444, 25.9702) (157.6147, 26.2453) (157.3793, 26.2453) knots 0 0 0 1 2 2 2
  spline S422 degree 2 poles (157.3793, 26.2453) (157.1382, 26.2453) (156.8659, 25.956) (156.8517, 25.7092) knots 0 0 0 1 2 2 2
  line L500 (156.8517, 25.7092) -> (157.8501, 25.7092)
  line L501 (161.5543, 24.05) -> (160.7261, 24.05)
  line L502 (160.7261, 24.05) -> (160.7261, 25.3575)
  spline S423 degree 2 poles (160.7261, 25.3575) (160.7261, 25.5192) (160.7006, 25.8369) (160.6665, 25.9106) knots 0 0 0 1 2 2 2
  spline S424 degree 2 poles (160.6665, 25.9106) (160.624, 26.0014) (160.4652, 26.078) (160.329, 26.078) knots 0 0 0 1 2 2 2
  spline S425 degree 2 poles (160.329, 26.078) (160.2297, 26.078) (160.0227, 26.0014) (159.9064, 25.9191) knots 0 0 0 1 2 2 2
  line L503 (159.9064, 25.9191) -> (159.9064, 24.05)
  line L504 (159.9064, 24.05) -> (159.0839, 24.05)
  line L505 (159.0839, 24.05) -> (159.0839, 26.6906)
  line L506 (159.0839, 26.6906) -> (159.9064, 26.6906)
  line L507 (159.9064, 26.6906) -> (159.9064, 26.3985)
  spline S426 degree 2 poles (159.9064, 26.3985) (160.1078, 26.5686) (160.4907, 26.7615) (160.7233, 26.7615) knots 0 0 0 1 2 2 2
  spline S427 degree 2 poles (160.7233, 26.7615) (161.126, 26.7615) (161.5543, 26.251) (161.5543, 25.7688) knots 0 0 0 1 2 2 2
  line L508 (161.5543, 25.7688) -> (161.5543, 24.05)
  spline S428 degree 2 poles (163.4575, 23.9791) (163.1313, 23.9791) (162.5895, 24.1436) (162.3882, 24.3138) knots 0 0 0 1 2 2 2
  spline S429 degree 2 poles (162.3882, 24.3138) (162.1925, 24.4868) (161.9712, 25.0058) (161.9712, 25.3575) knots 0 0 0 1 2 2 2
  spline S430 degree 2 poles (161.9712, 25.3575) (161.9712, 25.7376) (162.2095, 26.268) (162.4165, 26.4382) knots 0 0 0 1 2 2 2
  spline S431 degree 2 poles (162.4165, 26.4382) (162.6122, 26.6027) (163.1455, 26.7615) (163.4348, 26.7615) knots 0 0 0 1 2 2 2
  spline S432 degree 2 poles (163.4348, 26.7615) (163.6532, 26.7615) (164.09, 26.6594) (164.3112, 26.5488) knots 0 0 0 1 2 2 2
  line L509 (164.3112, 26.5488) -> (164.3112, 25.8454)
  line L510 (164.3112, 25.8454) -> (164.2062, 25.8454)
  spline S433 degree 2 poles (164.2062, 25.8454) (164.1552, 25.8936) (164.0134, 26.0071) (163.9283, 26.0524) knots 0 0 0 1 2 2 2
  spline S434 degree 2 poles (163.9283, 26.0524) (163.8375, 26.1035) (163.6135, 26.1716) (163.4745, 26.1716) knots 0 0 0 1 2 2 2
  spline S435 degree 2 poles (163.4745, 26.1716) (163.1596, 26.1716) (162.8136, 25.7319) (162.8136, 25.3575) knots 0 0 0 1 2 2 2
  spline S436 degree 2 poles (162.8136, 25.3575) (162.8136, 24.9605) (163.1823, 24.569) (163.4887, 24.569) knots 0 0 0 1 2 2 2
  spline S437 degree 2 poles (163.4887, 24.569) (163.6447, 24.569) (163.8772, 24.64) (163.9623, 24.691) knots 0 0 0 1 2 2 2
  spline S438 degree 2 poles (163.9623, 24.691) (164.0446, 24.7392) (164.1637, 24.847) (164.2062, 24.8895) knots 0 0 0 1 2 2 2
  line L511 (164.2062, 24.8895) -> (164.3112, 24.8895)
  line L512 (164.3112, 24.8895) -> (164.3112, 24.1833)
  spline S439 degree 2 poles (164.3112, 24.1833) (164.2403, 24.1521) (164.0559, 24.0727) (163.9595, 24.0472) knots 0 0 0 1 2 2 2
  spline S440 degree 2 poles (163.9595, 24.0472) (163.8404, 24.0131) (163.6305, 23.9791) (163.4575, 23.9791) knots 0 0 0 1 2 2 2
  line L513 (167.1645, 26.6906) -> (165.8343, 23.0828)
  line L514 (165.8343, 23.0828) -> (164.9494, 23.0828)
  line L515 (164.9494, 23.0828) -> (165.3493, 24.1152)
  line L516 (165.3493, 24.1152) -> (164.3821, 26.6906)
  line L517 (164.3821, 26.6906) -> (165.2443, 26.6906)
  line L518 (165.2443, 26.6906) -> (165.8002, 25.0342)
  line L519 (165.8002, 25.0342) -> (166.3193, 26.6906)
  line L520 (166.3193, 26.6906) -> (167.1645, 26.6906)
  spline S441 degree 2 poles (170.0235, 23.9876) (169.6207, 23.9876) (169.0138, 24.1436) (168.7528, 24.2571) knots 0 0 0 1 2 2 2
  line L521 (168.7528, 24.2571) -> (168.7528, 25.0909)
  line L522 (168.7528, 25.0909) -> (168.8323, 25.0909)
  spline S442 degree 2 poles (168.8323, 25.0909) (169.096, 24.8669) (169.7285, 24.6258) (170.0263, 24.6258) knots 0 0 0 1 2 2 2
  spline S443 degree 2 poles (170.0263, 24.6258) (170.1029, 24.6258) (170.3497, 24.6598) (170.4234, 24.6938) knots 0 0 0 1 2 2 2
  spline S444 degree 2 poles (170.4234, 24.6938) (170.5142, 24.7335) (170.6418, 24.8782) (170.6418, 24.9945) knots 0 0 0 1 2 2 2
  spline S445 degree 2 poles (170.6418, 24.9945) (170.6418, 25.1278) (170.4348, 25.2923) (170.2929, 25.3292) knots 0 0 0 1 2 2 2
  spline S446 degree 2 poles (170.2929, 25.3292) (170.1143, 25.3774) (169.7087, 25.4596) (169.53, 25.522) knots 0 0 0 1 2 2 2
  spline S447 degree 2 poles (169.53, 25.522) (169.1244, 25.6639) (168.7727, 26.1489) (168.7727, 26.5119) knots 0 0 0 1 2 2 2
  spline S448 degree 2 poles (168.7727, 26.5119) (168.7727, 27.0026) (169.6037, 27.6124) (170.2277, 27.6124) knots 0 0 0 1 2 2 2
  spline S449 degree 2 poles (170.2277, 27.6124) (170.5397, 27.6124) (171.158, 27.4848) (171.4019, 27.377) knots 0 0 0 1 2 2 2
  line L523 (171.4019, 27.377) -> (171.4019, 26.5771)
  line L524 (171.4019, 26.5771) -> (171.3254, 26.5771)
  spline S450 degree 2 poles (171.3254, 26.5771) (171.1297, 26.7445) (170.5681, 26.9742) (170.2731, 26.9742) knots 0 0 0 1 2 2 2
  spline S451 degree 2 poles (170.2731, 26.9742) (170.1568, 26.9742) (169.9753, 26.9402) (169.8732, 26.8948) knots 0 0 0 1 2 2 2
  spline S452 degree 2 poles (169.8732, 26.8948) (169.7909, 26.8579) (169.6718, 26.7105) (169.6718, 26.6197) knots 0 0 0 1 2 2 2
  spline S453 degree 2 poles (169.6718, 26.6197) (169.6718, 26.4835) (169.8618, 26.3276) (170.1341, 26.2652) knots 0 0 0 1 2 2 2
  spline S454 degree 2 poles (170.1341, 26.2652) (170.31, 26.2254) (170.6361, 26.1489) (170.8233, 26.0836) knots 0 0 0 1 2 2 2
  spline S455 degree 2 poles (170.8233, 26.0836) (171.1864, 25.9503) (171.5409, 25.5079) (171.5409, 25.1448) knots 0 0 0 1 2 2 2
  spline S456 degree 2 poles (171.5409, 25.1448) (171.5409, 24.6229) (170.7212, 23.9876) (170.0235, 23.9876) knots 0 0 0 1 2 2 2
  spline S457 degree 2 poles (172.9534, 23.9989) (172.4514, 23.9989) (171.9919, 24.413) (171.9919, 24.8839) knots 0 0 0 1 2 2 2
  line L525 (171.9919, 24.8839) -> (171.9919, 26.1177)
  line L526 (171.9919, 26.1177) -> (171.6771, 26.1177)
  line L527 (171.6771, 26.1177) -> (171.6771, 26.6906)
  line L528 (171.6771, 26.6906) -> (171.9919, 26.6906)
  line L529 (171.9919, 26.6906) -> (171.9919, 27.4451)
  line L530 (171.9919, 27.4451) -> (172.8144, 27.4451)
  line L531 (172.8144, 27.4451) -> (172.8144, 26.6906)
  line L532 (172.8144, 26.6906) -> (173.6086, 26.6906)
  line L533 (173.6086, 26.6906) -> (173.6086, 26.1177)
  line L534 (173.6086, 26.1177) -> (172.8144, 26.1177)
  line L535 (172.8144, 26.1177) -> (172.8144, 25.1788)
  spline S458 degree 2 poles (172.8144, 25.1788) (172.8144, 25.0399) (172.8201, 24.8328) (172.8541, 24.7506) knots 0 0 0 1 2 2 2
  spline S459 degree 2 poles (172.8541, 24.7506) (172.8882, 24.6683) (173.0555, 24.5719) (173.2143, 24.5719) knots 0 0 0 1 2 2 2
  spline S460 degree 2 poles (173.2143, 24.5719) (173.2824, 24.5719) (173.4951, 24.6286) (173.5377, 24.6513) knots 0 0 0 1 2 2 2
  line L536 (173.5377, 24.6513) -> (173.6086, 24.6513)
  line L537 (173.6086, 24.6513) -> (173.6086, 24.0727)
  spline S461 degree 2 poles (173.6086, 24.0727) (173.4753, 24.0387) (173.1746, 23.9989) (172.9534, 23.9989) knots 0 0 0 1 2 2 2
  spline S462 degree 2 poles (176.4761, 25.3689) (176.4761, 24.7165) (175.7642, 23.9677) (175.1147, 23.9677) knots 0 0 0 1 2 2 2
  spline S463 degree 2 poles (175.1147, 23.9677) (174.468, 23.9677) (173.7504, 24.7165) (173.7504, 25.3689) knots 0 0 0 1 2 2 2
  spline S464 degree 2 poles (173.7504, 25.3689) (173.7504, 26.0269) (174.468, 26.7729) (175.1147, 26.7729) knots 0 0 0 1 2 2 2
  spline S465 degree 2 poles (175.1147, 26.7729) (175.7613, 26.7729) (176.4761, 26.0241) (176.4761, 25.3689) knots 0 0 0 1 2 2 2
  spline S466 degree 2 poles (175.6337, 25.3632) (175.6337, 25.5986) (175.5571, 25.9135) (175.4891, 26.0071) knots 0 0 0 1 2 2 2
  spline S467 degree 2 poles (175.4891, 26.0071) (175.4153, 26.1063) (175.231, 26.1829) (175.1147, 26.1829) knots 0 0 0 1 2 2 2
  spline S468 degree 2 poles (175.1147, 26.1829) (175.0012, 26.1829) (174.8225, 26.1148) (174.7488, 26.0184) knots 0 0 0 1 2 2 2
  spline S469 degree 2 poles (174.7488, 26.0184) (174.6779, 25.9276) (174.5928, 25.6071) (174.5928, 25.3632) knots 0 0 0 1 2 2 2
  spline S470 degree 2 poles (174.5928, 25.3632) (174.5928, 25.1221) (174.6722, 24.8243) (174.7374, 24.7335) knots 0 0 0 1 2 2 2
  spline S471 degree 2 poles (174.7374, 24.7335) (174.8027, 24.6428) (175.0012, 24.5577) (175.1203, 24.5577) knots 0 0 0 1 2 2 2
  spline S472 degree 2 poles (175.1203, 24.5577) (175.2196, 24.5577) (175.4238, 24.6428) (175.4862, 24.7279) knots 0 0 0 1 2 2 2
  spline S473 degree 2 poles (175.4862, 24.7279) (175.5571, 24.8271) (175.6337, 25.1136) (175.6337, 25.3632) knots 0 0 0 1 2 2 2
  spline S474 degree 2 poles (179.4996, 25.4058) (179.4996, 24.7733) (178.8586, 23.9989) (178.3878, 23.9989) knots 0 0 0 1 2 2 2
  spline S475 degree 2 poles (178.3878, 23.9989) (178.1921, 23.9989) (177.8999, 24.0869) (177.7354, 24.1833) knots 0 0 0 1 2 2 2
  line L538 (177.7354, 24.1833) -> (177.7354, 23.0828)
  line L539 (177.7354, 23.0828) -> (176.9129, 23.0828)
  line L540 (176.9129, 23.0828) -> (176.9129, 26.6906)
  line L541 (176.9129, 26.6906) -> (177.7354, 26.6906)
  line L542 (177.7354, 26.6906) -> (177.7354, 26.4126)
  spline S476 degree 2 poles (177.7354, 26.4126) (177.9169, 26.5686) (178.2913, 26.7615) (178.5381, 26.7615) knots 0 0 0 1 2 2 2
  spline S477 degree 2 poles (178.5381, 26.7615) (178.9976, 26.7615) (179.4996, 26.0326) (179.4996, 25.4058) knots 0 0 0 1 2 2 2
  spline S478 degree 2 poles (178.6572, 25.3887) (178.6572, 25.7745) (178.419, 26.1205) (178.1694, 26.1205) knots 0 0 0 1 2 2 2
  spline S479 degree 2 poles (178.1694, 26.1205) (178.0588, 26.1205) (177.8404, 26.0496) (177.7354, 25.9787) knots 0 0 0 1 2 2 2
  line L543 (177.7354, 25.9787) -> (177.7354, 24.6541)
  spline S480 degree 2 poles (177.7354, 24.6541) (177.8006, 24.6258) (177.9595, 24.6031) (178.0673, 24.6031) knots 0 0 0 1 2 2 2
  spline S481 degree 2 poles (178.0673, 24.6031) (178.3651, 24.6031) (178.6572, 24.9945) (178.6572, 25.3887) knots 0 0 0 1 2 2 2
  point P0 (0, 0)
  point P1 (-175, 0)
  point P2 (-175, 0)
  point P3 (-180, 21.55)
  point P4 (-110, 0)
  point P5 (-115, 21.55)
  point P6 (-45, 0)
  point P7 (-50, 21.55)
  point P8 (15, 21.55)
  point P9 (152.0226, 0.85)
  point P10 (160, 0)
  dimension "d15" = 23.6
  dimension "d16" = 3.1
  dimension "d17" = 19
  dimension "d18" = 24
  dimension "d19" = 175
  dimension "d20" = 10
  dimension "d21" = 10
  dimension "d22" = 10
  dimension "d23" = 23.52
  dimension "d24" = 23.52
  dimension "d25" = 3.1
  dimension "d26" = 2.5
  dimension "d27" = 41.521
  dimension "d28" = 110
  dimension "d29" = 10
  dimension "d30" = 10
  dimension "d31" = 11.2
  dimension "d32" = 16.66
  dimension "d33" = 16.66
  dimension "d34" = 3.1
  dimension "d35" = 2.5
  dimension "d36" = 28.2
  dimension "d37" = 45
  dimension "d38" = 18
  dimension "d39" = 8.2
  dimension "d40" = 2.1
  dimension "d41" = 2.1
  dimension "d42" = 18
  dimension "d43" = 8.2
  dimension "d44" = 2.1
  dimension "d45" = 2.1
  dimension "d46" = 18
  dimension "d47" = 8.2
  dimension "d48" = 2.1
  dimension "d49" = 2.1
  dimension "d50" = 20
  dimension "d53" = 8
  dimension "d55" = 17
  dimension "d58" = 25
  dimension "d59" = 5
  dimension "d60" = 10
  dimension "d61" = 5
  dimension "d62" = 5
  dimension "d63" = 5
  dimension "d64" = 5
  dimension "d65" = 5
  dimension "d66" = 5
  dimension "d67" = 5
  dimension "d70" = 16
  dimension "d71" = 15
  dimension "d72" = 1.7
  dimension "d73" = 40
  dimension "d74" = 40
  dimension "d75" = 25
  dimension "d76" = 60
  dimension "d77" = 5
  constraints: 146 end point, 36 point on circle, 34 midpoint, 29 point on line, 28 horizontal, 23 centre point, 22 parallel, 16 collinear, 16 tangent, 14 perpendicular, 9 equal radius, 6 coincident, 6 vertical, 11 other
  measures "d15" diameter of A12
  measures "d16" diameter of A13
  measures "d17" distance of L13.end L14.end
  measures "d18" distance of L14.end L12.start
  measures "d19" distance of point (0, 0) point (-175, 0)
  measures "d20" angle of L25 L21
  measures "d21" angle of L23 L19
  measures "d22" distance between parallel lines of L20 L18
  measures "d23" distance from line of A15.centre L26
  measures "d24" distance from line of A16.centre L26
  measures "d25" diameter of A15
  measures "d26" radius of A17
  measures "d27" distance of L19.start L21.end
  measures "d28" distance from line of L26 point (0, 0)
  measures "d29" angle of L35 L31
  measures "d30" angle of L33 L29
  measures "d31" distance between parallel lines of L30 L28
  measures "d32" distance from line of A21.centre L36
  measures "d33" distance from line of A22.centre L36
  measures "d34" diameter of A21
  measures "d35" radius of A23
  measures "d36" distance of L29.start L31.end